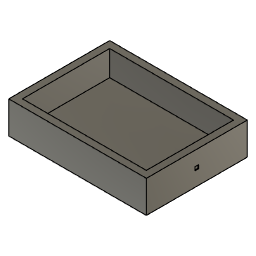
NRC_2020_Body (Autodesk Fusion 360 design; units mm, degrees)
Autodesk Fusion 360 part; units mm, degrees
sketch "Sketch1" plane through (0, 0, 0) normal (0, 0, 1) x (1, 0, 0) in component "bottom"
  line L0 (150, 110) -> (-150, 110)
  line L1 (-150, 110) -> (-150, -110)
  line L2 (-150, -110) -> (150, -110)
  line L3 (150, -110) -> (150, 110)
  line L4 (150, 110) -> (-150, -110) construction
  line L5 (-150, 110) -> (150, -110) construction
  dimension "d1" = 300
  dimension "d2" = 220
  constraint perpendicular L0 L1
  constraint parallel L0 L2
  constraint parallel L1 L3
  constraint horizontal L0
  constraint coincident L4 origin
  constraint coincident L5 origin
  measures "d1" distance of L1.end L2.end
  measures "d2" distance of L0.end L1.end
extrude "Extrude1" add sketch "Sketch1" along normal blind 70 in component "bottom"
sketch "Sketch2" plane through (150, 0, 0) normal (1, 0, 0) x (0, 1, 0) in component "bottom"
  line L0 (-110, 0) -> (110, 0)
  line L1 (110, 0) -> (110, 70)
  line L2 (110, 70) -> (-110, 70)
  line L3 (-110, 70) -> (-110, 0)
  line L4 (-12.5, 47.5) -> (12.5, 47.5)
  line L5 (12.5, 47.5) -> (12.5, 22.5)
  line L6 (12.5, 22.5) -> (-12.5, 22.5)
  line L7 (-12.5, 22.5) -> (-12.5, 47.5)
  line L8 (-12.5, 47.5) -> (12.5, 22.5) construction
  line L9 (12.5, 47.5) -> (-12.5, 22.5) construction
  line L10 (3.9, 31.1) -> (-3.9, 31.1)
  line L11 (-3.9, 31.1) -> (-3.9, 38.9)
  line L12 (-3.9, 38.9) -> (3.9, 38.9)
  line L13 (3.9, 38.9) -> (3.9, 31.1)
  point P0 (0, 35)
  dimension "d5" = 25
  dimension "d6" = 25
  dimension "d7" = 8.6
  constraint perpendicular L4 L5
  constraint parallel L4 L6
  constraint parallel L5 L7
  constraint horizontal L4
  constraint coincident L8 P0
  constraint coincident L9 P0
  measures "d5" distance of L5.end L6.end
  measures "d6" distance of L4.end L5.end
extrude "Extrude2" cut sketch "Sketch2" against normal blind 1.6 contours L10 L11 L12 L13 in component "bottom"
sketch "Sketch3" plane through (0, 0, 70) normal (0, 0, 1) x (-1, 0, 0) in component "bottom"
  line L0 (-150, 110) -> (-150, -110)
  line L1 (-150, -110) -> (150, -110)
  line L2 (150, -110) -> (150, 110)
  line L3 (150, 110) -> (-150, 110)
  line L4 (135, 95) -> (-135, 95)
  line L5 (-135, 95) -> (-135, -95)
  line L6 (-135, -95) -> (135, -95)
  line L7 (135, -95) -> (135, 95)
  dimension "d10" = -15
extrude "Extrude3" cut sketch "Sketch3" against normal up to surface (55 mm away) contours L4 L5 L6 L7 in component "bottom"
component "bottom" placed x (1, 0, 0) y (0, 1, 0) z (0, 0, 1) at (0, 0, 0)
component "top" placed x (1, 0, 0) y (0, 1, 0) z (0, 0, 1) at (0, 0, 0)
